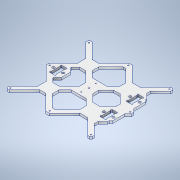
# Autodesk Inventor part: FROG
Saved by Autodesk Inventor 2023 (Build 270158000, 158)
## iProperties
Created: 2019-06-17
Part Number: FROG
Material: Aluminum 6061
Document SubType Name: Modeling
Designer: pepd9
Density: 2.7 g/cm^3
Appearance: Aluminum - Flat
Description: ALUM FROG
Author: pepd9
Autodesk Inventor part; units mm, degrees
ref_plane "YZ Plane" through (0, 0, 0) normal (1, 0, 0) x (0, 1, 0)
ref_plane "XZ Plane" through (0, 0, 0) normal (0, 1, 0) x (-1, 0, 0)
ref_plane "XY Plane" through (0, 0, 0) normal (0, 0, 1) x (1, 0, 0)
sketch "Sketch1" plane through (0, 0, 0) normal (0, 1, 0) x (-1, 0, 0)
  line L0 (-116, -3.7391) -> (-98.5, -21.2391)
  line L1 (-98.5, -21.2391) -> (-98.5, -52.5)
  line L2 (-98.5, -52.5) -> (-89, -62)
  line L3 (-89, -62) -> (-89, -75.5147)
  line L4 (-89, -75.5147) -> (-116, -102.5147)
  line L5 (-116, -102.5147) -> (-116, -107.4852)
  line L6 (-116, -107.4852) -> (-112.4852, -111)
  line L7 (-112.4852, -111) -> (-107.5147, -111)
  line L8 (-107.5147, -111) -> (-66.5147, -70)
  line L9 (-66.5147, -70) -> (-45.4001, -70)
  line L10 (-45.4001, -70) -> (-4.4001, -111)
  line L11 (-4.4001, -111) -> (4.4001, -111)
  line L12 (4.4001, -111) -> (45.4001, -70)
  line L13 (45.4001, -70) -> (61.5147, -70)
  line L14 (61.5147, -70) -> (102.5147, -111)
  line L15 (102.5147, -111) -> (107.4852, -111)
  line L16 (107.4852, -111) -> (111, -107.4852)
  line L17 (111, -107.4852) -> (111, -102.5147)
  line L18 (111, -102.5147) -> (73, -64.5147)
  line L19 (73, -64.5147) -> (73, -41.667)
  line L20 (73, -41.667) -> (111, -3.667)
  line L21 (111, -3.667) -> (111, 3.667)
  line L22 (111, 3.667) -> (73, 41.667)
  line L23 (73, 41.667) -> (73, 64.5147)
  line L24 (73, 64.5147) -> (111, 102.5147)
  line L25 (111, 102.5147) -> (111, 107.4852)
  line L26 (111, 107.4852) -> (107.4852, 111)
  line L27 (107.4852, 111) -> (102.5147, 111)
  line L28 (102.5147, 111) -> (61.5147, 70)
  line L29 (61.5147, 70) -> (45.4001, 70)
  line L30 (45.4001, 70) -> (4.4001, 111)
  line L31 (4.4001, 111) -> (-4.4001, 111)
  line L32 (-4.4001, 111) -> (-45.4001, 70)
  line L33 (-45.4001, 70) -> (-66.5147, 70)
  line L34 (-66.5147, 70) -> (-107.5147, 111)
  line L35 (-107.5147, 111) -> (-112.4852, 111)
  line L36 (-112.4852, 111) -> (-116, 107.4852)
  line L37 (-116, 107.4852) -> (-116, 102.5147)
  line L38 (-116, 102.5147) -> (-89, 75.5147)
  line L39 (-89, 75.5147) -> (-89, 62)
  line L40 (-89, 62) -> (-98.5, 52.5)
  line L41 (-98.5, 52.5) -> (-98.5, 21.2391)
  line L42 (-98.5, 21.2391) -> (-116, 3.7391)
  line L43 (-116, -3.7391) -> (-116, 3.7391)
  line L44 (-38.023, -28) -> (-18, -7.977)
  line L45 (-55, -28) -> (-38.023, -28)
  line L46 (-78.5, -4.5) -> (-55, -28)
  line L47 (-78.5, -4.5) -> (-78.5, 4.5)
  line L48 (-55, 28) -> (-78.5, 4.5)
  line L49 (-38.023, 28) -> (-55, 28)
  line L50 (-18, 7.977) -> (-38.023, 28)
  line L51 (-18, -7.977) -> (-18, 7.977)
  circle A0 centre (1.5, -19.5) radius 1.5
  circle A1 centre (1.5, 19.5) radius 1.5
  circle A2 centre (-110, 105) radius 1.5
  circle A3 centre (-93.5, 35) radius 1.6
  circle A4 centre (-93.5, -35) radius 1.6
  circle A5 centre (-73.5, 35) radius 1.6
  circle A6 centre (-73.5, -35) radius 1.6
  circle A7 centre (96.5, 0) radius 1.6
  circle A8 centre (76.5, 0) radius 1.6
  circle A9 centre (105, 0) radius 1.5
  circle A10 centre (0, 0) radius 1.5
  circle A11 centre (-110, 0) radius 1.5
  circle A12 centre (105, -105) radius 1.5
  circle A13 centre (-110, -105) radius 1.5
  circle A14 centre (105, 105) radius 1.5
  circle A15 centre (0, -105) radius 1.5
  circle A16 centre (0, 105) radius 1.5
  arc A17 (-89.1, -42.25) -> (-89.1, -48.25) centre (-89.1, -45.25) ccw
  line L52 (-89.1, -42.25) -> (-89, -42.25)
  line L53 (-88.5, -41.75) -> (-89, -42.25)
  line L54 (-88.5, -41.75) -> (-88.5, -28.25)
  line L55 (-89, -27.75) -> (-88.5, -28.25)
  line L56 (-89.1, -27.75) -> (-89, -27.75)
  arc A18 (-89.1, -21.75) -> (-89.1, -27.75) centre (-89.1, -24.75) ccw
  line L57 (-89.1, -21.75) -> (-77.9, -21.75)
  arc A19 (-77.9, -27.75) -> (-77.9, -21.75) centre (-77.9, -24.75) ccw
  line L58 (-77.9, -27.75) -> (-78, -27.75)
  line L59 (-78, -27.75) -> (-78.5, -28.25)
  line L60 (-78.5, -41.75) -> (-78.5, -28.25)
  line L61 (-78.5, -41.75) -> (-78, -42.25)
  line L62 (-77.9, -42.25) -> (-78, -42.25)
  arc A20 (-77.9, -48.25) -> (-77.9, -42.25) centre (-77.9, -45.25) ccw
  line L63 (-89.1, -48.25) -> (-77.9, -48.25)
  arc A21 (80.9, -7.25) -> (80.9, -13.25) centre (80.9, -10.25) ccw
  line L64 (80.9, -7.25) -> (81, -7.25)
  line L65 (81.5, -6.75) -> (81, -7.25)
  line L66 (81.5, -6.75) -> (81.5, 6.75)
  line L67 (81, 7.25) -> (81.5, 6.75)
  line L68 (80.9, 7.25) -> (81, 7.25)
  arc A22 (80.9, 13.25) -> (80.9, 7.25) centre (80.9, 10.25) ccw
  line L69 (80.9, 13.25) -> (92.1, 13.25)
  arc A23 (92.1, 7.25) -> (92.1, 13.25) centre (92.1, 10.25) ccw
  line L70 (92.1, 7.25) -> (92, 7.25)
  line L71 (92, 7.25) -> (91.5, 6.75)
  line L72 (91.5, -6.75) -> (91.5, 6.75)
  line L73 (91.5, -6.75) -> (92, -7.25)
  line L74 (92.1, -7.25) -> (92, -7.25)
  arc A24 (92.1, -13.25) -> (92.1, -7.25) centre (92.1, -10.25) ccw
  line L75 (80.9, -13.25) -> (92.1, -13.25)
  arc A25 (-89.1, 27.75) -> (-89.1, 21.75) centre (-89.1, 24.75) ccw
  line L76 (-89.1, 27.75) -> (-89, 27.75)
  line L77 (-88.5, 28.25) -> (-89, 27.75)
  line L78 (-88.5, 28.25) -> (-88.5, 41.75)
  line L79 (-89, 42.25) -> (-88.5, 41.75)
  line L80 (-89.1, 42.25) -> (-89, 42.25)
  arc A26 (-89.1, 48.25) -> (-89.1, 42.25) centre (-89.1, 45.25) ccw
  line L81 (-89.1, 48.25) -> (-77.9, 48.25)
  arc A27 (-77.9, 42.25) -> (-77.9, 48.25) centre (-77.9, 45.25) ccw
  line L82 (-77.9, 42.25) -> (-78, 42.25)
  line L83 (-78, 42.25) -> (-78.5, 41.75)
  line L84 (-78.5, 28.25) -> (-78.5, 41.75)
  line L85 (-78.5, 28.25) -> (-78, 27.75)
  line L86 (-77.9, 27.75) -> (-78, 27.75)
  arc A28 (-77.9, 21.75) -> (-77.9, 27.75) centre (-77.9, 24.75) ccw
  line L87 (-89.1, 21.75) -> (-77.9, 21.75)
  line L88 (3.6826, 94.747) -> (-3.6826, 94.7332)
  line L89 (36, 62.4296) -> (3.6826, 94.747)
  line L90 (36, 44.4853) -> (36, 62.4296)
  line L91 (19.5147, 28) -> (36, 44.4853)
  line L92 (-20.4337, 28) -> (19.5147, 28)
  line L93 (-37, 44.5663) -> (-20.4337, 28)
  line L94 (-37, 61.4158) -> (-37, 44.5663)
  line L95 (-3.6826, 94.7332) -> (-37, 61.4158)
  line L96 (-3.6826, -94.7332) -> (-37, -61.4158)
  line L97 (-37, -61.4158) -> (-37, -44.5663)
  line L98 (-37, -44.5663) -> (-20.4337, -28)
  line L99 (-20.4337, -28) -> (19.5147, -28)
  line L100 (19.5147, -28) -> (36, -44.4853)
  line L101 (36, -44.4853) -> (36, -62.4296)
  line L102 (36, -62.4296) -> (3.6826, -94.747)
  line L103 (3.6826, -94.747) -> (-3.6826, -94.7332)
  line L104 (17, -8.5147) -> (17, 8.5147)
  line L105 (17, 8.5147) -> (44.0147, 35.5294)
  line L106 (44.0147, 35.5294) -> (60.9853, 35.5294)
  line L107 (60.9853, 35.5294) -> (71.5, 25.0147)
  line L108 (71.5, -25.0147) -> (71.5, 25.0147)
  line L109 (71.5, -25.0147) -> (60.9853, -35.5294)
  line L110 (60.9853, -35.5294) -> (44.0147, -35.5294)
  line L111 (44.0147, -35.5294) -> (17, -8.5147)
  line L112 (-116, -111) -> (111, -111)
  line L113 (111, -111) -> (111, 111)
  line L114 (111, 111) -> (-116, 111)
  line L115 (-116, 111) -> (-116, -111)
  constraints: 232 end point, 29 centre point, 24 point on circle, 2 parallel, 1 horizontal, 1 perpendicular
sketch "Sketch2" plane through (0, 0, 0) normal (0, 1, 0) x (-1, 0, 0)
  circle A0 centre (105, -105) radius 1.5 projected
  circle A1 centre (0, -105) radius 1.5 projected
  circle A2 centre (-110, -105) radius 1.5 projected
  circle A3 centre (-110, 0) radius 1.5 projected
  circle A4 centre (0, 0) radius 1.5 projected
  circle A5 centre (105, 0) radius 1.5 projected
  circle A6 centre (105, 105) radius 1.5 projected
  circle A7 centre (-110, 105) radius 1.5 projected
  circle A8 centre (0, 105) radius 1.5 projected
  line L0 (102.5147, -111) -> (107.4852, -111) projected
  line L1 (111, -107.4852) -> (111, -102.5147) projected
  line L2 (-112.4852, -111) -> (-107.5147, -111) projected
  line L3 (-116, -102.5147) -> (-116, -107.4852) projected
  line L4 (-116, 107.4852) -> (-116, 102.5147) projected
  line L5 (-107.5147, 111) -> (-112.4852, 111) projected
  line L6 (107.4852, 111) -> (102.5147, 111) projected
  line L7 (111, 102.5147) -> (111, 107.4852) projected
  line L8 (111, 111) -> (-116, 111)
  line L9 (-116, 111) -> (-116, -111)
  line L10 (-116, -111) -> (111, -111)
  line L11 (111, -111) -> (111, 111)
  constraints: 8 end point, 2 parallel, 1 horizontal, 1 perpendicular
extrude "Extrusion1" add sketch "Sketch2" along normal blind 6.35
ref_plane "Work Plane1" through (2.5, 0, 111) normal (1, 0, 0) x (0, 0, -1)
sketch "Sketch6" plane through (0, 6.35, 0) normal (0, 1, 0) x (1, 0, 0)
  line L0 (73.5, -35) -> (93.5, -35)
  line L1 (73.5, 35) -> (93.5, 35)
  line L2 (80.75, 20.5) -> (94.25, 20.5)
  line L3 (94.25, 20.5) -> (94.25, 49.5)
  line L4 (94.25, 49.5) -> (80.75, 49.5)
  line L5 (80.75, 49.5) -> (80.75, 20.5)
  line L6 (80.75, 20.5) -> (94.25, 49.5) construction
  line L7 (94.25, 20.5) -> (80.75, 49.5) construction
  line L8 (80.75, -49.5) -> (94.25, -49.5)
  line L9 (94.25, -49.5) -> (94.25, -20.5)
  line L10 (94.25, -20.5) -> (80.75, -20.5)
  line L11 (80.75, -20.5) -> (80.75, -49.5)
  line L12 (80.75, -49.5) -> (94.25, -20.5) construction
  line L13 (94.25, -49.5) -> (80.75, -20.5) construction
  line L14 (87.5, -199.2866) -> (87.5, 58.81)
  line L15 (87.5, 0) -> (-102.0147, 0)
  line L16 (-75.75, 14.5) -> (-89.25, 14.5)
  line L17 (-89.25, 14.5) -> (-89.25, -14.5)
  line L18 (-89.25, -14.5) -> (-75.75, -14.5)
  line L19 (-75.75, -14.5) -> (-75.75, 14.5)
  line L20 (-75.75, 14.5) -> (-89.25, -14.5) construction
  line L21 (-89.25, 14.5) -> (-75.75, -14.5) construction
  point P0 (0, 0)
  point P1 (-82.5, 0)
  dimension "d16" = 13.5
  dimension "d17" = 29
  dimension "d18" = 13.5
  dimension "d19" = 29
  dimension "d39" = 6.75
  dimension "d40" = 6.75
  dimension "d67" = 87.5
  dimension "d68" = 13.5
  dimension "d69" = 29
  dimension "d70" = 170
  dimension "d76" = 14.5
  dimension "d77" = 14.5
  constraints: 44 end point, 6 horizontal, 6 parallel, 3 perpendicular, 2 midpoint, 2 point on line, 1 vertical
  measures "d16" distance of L4.end L3.end
  measures "d17" distance of L3.end L2.end
  measures "d18" distance of L10.end L9.end
  measures "d19" distance of L9.end L8.end
  measures "d39" distance between parallel lines of L14 L3
  measures "d40" distance between parallel lines of L14 L9
  measures "d67" distance from line of L14 point (0, 0)
  measures "d68" distance of L18.end L17.end
  measures "d69" distance of L17.end L16.end
  measures "d70" distance from line of L14 point (-82.5, 0)
  measures "d76" distance between parallel lines of L0 L8
  measures "d77" distance between parallel lines of L1 L4
extrude "Extrusion5" cut sketch "Sketch6" against normal through all
sketch "Sketch10" plane through (0, 6.35, 0) normal (0, 1, 0) x (1, 0, 0)
  line L0 (116, 111) -> (-111, 111) projected
  line L1 (-111, 111) -> (-111, -111) projected
  line L2 (-111, -111) -> (116, -111) projected
  line L3 (116, -111) -> (116, 111) projected
  circle A0 centre (0, -105) radius 1.5 projected
  circle A1 centre (-105, 105) radius 1.5 projected
  circle A2 centre (0, 105) radius 1.5 projected
  circle A3 centre (110, 105) radius 1.5 projected
  circle A4 centre (110, 0) radius 1.5 projected
  circle A5 centre (0, 0) radius 1.5 projected
  circle A6 centre (-105, 0) radius 1.5 projected
  circle A7 centre (-105, -105) radius 1.5 projected
  circle A8 centre (110, -105) radius 1.5 projected
  line L4 (94.25, -20.5) -> (94.25, -49.5) projected
  line L5 (80.75, -49.5) -> (80.75, -20.5) projected
  line L6 (80.75, 20.5) -> (80.75, 49.5) projected
  line L7 (94.25, 49.5) -> (94.25, 20.5) projected
  line L8 (80.75, -20.5) -> (94.25, -20.5) projected
  line L9 (94.25, -49.5) -> (80.75, -49.5) projected
  line L10 (80.75, 49.5) -> (94.25, 49.5) projected
  line L11 (94.25, 20.5) -> (80.75, 20.5) projected
extrude "Extrusion7" cut sketch "Sketch1" along normal blind 10 contours A0 | A1
sketch "Sketch13" plane through (0, 0, 0) normal (0, -1, 0) x (1, 0, 0)
  point P0 (0, 0)
extrude "Extrusion8" cut sketch "Sketch1" along normal blind 10 contours L6 L112 L115 | L115 L114 L36 | L8 L9 L10 L112 | L114 L32 L33 L34 | L12 L13 L14 L112 | L114 L28 L29 L30 | L16 L113 L112 | L114 L113 L26 | L18 L19 L20 L113 | L113 L22 L23 L24 | A0 | A1 | A2 | A9 | A10 | A11 | A12 | A13 | A14 | A15 | A16 | L89 L90 L91 L92 L93 L94 L95 L88 | L96 L97 L98 L99 L100 L101 L102 L103
sketch "Sketch14" plane through (0, 0, 0) normal (0, -1, 0) x (1, 0, 0)
  line L0 (89, -62) -> (89, -75.5147) projected
  line L1 (116, 102.5147) -> (89, 75.5147)
  line L2 (89, 75.5147) -> (89, 62)
  line L3 (89, 62) -> (107.1558, 43.8442)
  line L4 (107.1558, 43.8442) -> (107.1558, 12.5833)
  line L5 (98.5, 21.2391) -> (116, 3.7391) projected
  line L6 (107.1558, 12.5833) -> (116, 3.7391)
  line L7 (116, 107.4852) -> (116, -107.4852) projected
  line L8 (116, 0) -> (13.4853, 0)
  line L9 (116, -102.5147) -> (89, -75.5147)
  line L10 (89, -75.5147) -> (89, -62)
  line L11 (89, -62) -> (107.1558, -43.8442)
  line L12 (107.1558, -43.8442) -> (107.1558, -12.5833)
  line L13 (98.5, -21.2391) -> (116, -3.7391)
  line L14 (107.1558, -12.5833) -> (116, -3.7391)
  line L15 (116, 102.5147) -> (116, -102.5147)
  line L16 (55, 28) -> (78.5, 4.5) projected
  line L17 (38.023, 28) -> (55, 28) projected
  line L18 (18, 7.977) -> (38.023, 28) projected
  line L19 (18, -7.977) -> (18, 7.977) projected
  line L20 (38.023, -28) -> (18, -7.977) projected
  line L21 (55, -28) -> (38.023, -28) projected
  line L22 (78.5, -4.5) -> (55, -28) projected
  line L23 (78.5, -4.5) -> (78.5, 4.5) projected
  point P0 (0, 0)
  constraints: 26 end point, 3 symmetric about line, 2 point on line, 1 collinear, 1 horizontal, 1 midpoint, 1 parallel, 1 vertical
extrude "Extrusion9" cut sketch "Sketch14" against normal blind 10
sketch "Sketch15" plane through (0, 0, 0) normal (0, -1, 0) x (1, 0, 0)
  line L0 (-17, -8.5147) -> (-17, 8.5147) projected
  line L1 (-17, 8.5147) -> (-44.0147, 35.5294) projected
  line L2 (-44.0147, 35.5294) -> (-60.9853, 35.5294) projected
  line L3 (-60.9853, 35.5294) -> (-71.5, 25.0147) projected
  line L4 (-44.0147, -35.5294) -> (-17, -8.5147) projected
  line L5 (-60.9853, -35.5294) -> (-44.0147, -35.5294) projected
  line L6 (107.1558, -12.5833) -> (116, -3.7391) projected
  line L7 (116, 3.7391) -> (116, -3.7391) projected
  line L8 (116, 3.7391) -> (107.1558, 12.5833) projected
  line L9 (107.1558, 12.5833) -> (107.1558, 43.8442) projected
  line L10 (107.1558, 43.8442) -> (89, 62) projected
  line L11 (89, 62) -> (89, 75.5147) projected
  line L12 (89, 75.5147) -> (116, 102.5147) projected
  line L13 (116, 107.4852) -> (116, 102.5147) projected
  line L14 (116, 107.4852) -> (112.4852, 111) projected
  line L15 (107.5147, 111) -> (112.4852, 111) projected
  line L16 (107.5147, 111) -> (66.5147, 70) projected
  line L17 (66.5147, 70) -> (45.4001, 70) projected
  line L18 (45.4001, 70) -> (4.4001, 111) projected
  line L19 (-4.4001, 111) -> (4.4001, 111) projected
  line L20 (-4.4001, 111) -> (-45.4001, 70) projected
  line L21 (-45.4001, 70) -> (-61.5147, 70) projected
  line L22 (-61.5147, 70) -> (-102.5147, 111) projected
  line L23 (-107.4852, 111) -> (-102.5147, 111) projected
  line L24 (-107.4852, 111) -> (-111, 107.4852) projected
  line L25 (-111, 102.5147) -> (-111, 107.4852) projected
  line L26 (-111, 102.5147) -> (-73, 64.5147) projected
  line L27 (-73, 64.5147) -> (-73, 41.667) projected
  line L28 (-73, 41.667) -> (-111, 3.667) projected
  line L29 (-111, -3.667) -> (-111, 3.667) projected
  line L30 (-111, -3.667) -> (-73, -41.667) projected
  line L31 (-73, -41.667) -> (-73, -64.5147) projected
  line L32 (-73, -64.5147) -> (-111, -102.5147) projected
  line L33 (-111, -107.4852) -> (-111, -102.5147) projected
  line L34 (-111, -107.4852) -> (-107.4852, -111) projected
  line L35 (-102.5147, -111) -> (-107.4852, -111) projected
  line L36 (-102.5147, -111) -> (-61.5147, -70) projected
  line L37 (-61.5147, -70) -> (-45.4001, -70) projected
  line L38 (-45.4001, -70) -> (-4.4001, -111) projected
  line L39 (4.4001, -111) -> (-4.4001, -111) projected
  line L40 (4.4001, -111) -> (45.4001, -70) projected
  line L41 (45.4001, -70) -> (66.5147, -70) projected
  line L42 (66.5147, -70) -> (107.5147, -111) projected
  line L43 (112.4852, -111) -> (107.5147, -111) projected
  line L44 (112.4852, -111) -> (116, -107.4852) projected
  line L45 (116, -102.5147) -> (116, -107.4852) projected
  line L46 (116, -102.5147) -> (89, -75.5147) projected
  line L47 (89, -75.5147) -> (89, -62) projected
  line L48 (89, -62) -> (107.1558, -43.8442) projected
  line L49 (107.1558, -43.8442) -> (107.1558, -12.5833) projected
  line L50 (18, -7.977) -> (18, 7.977) projected
  line L51 (18, 7.977) -> (38.023, 28) projected
  line L52 (38.023, 28) -> (55, 28) projected
  line L53 (55, 28) -> (78.5, 4.5) projected
  line L54 (78.5, 4.5) -> (78.5, -4.5) projected
  line L55 (78.5, -4.5) -> (55, -28) projected
  line L56 (55, -28) -> (38.023, -28) projected
  line L57 (38.023, -28) -> (18, -7.977) projected
  line L58 (94.25, -20.5) -> (94.25, -49.5) projected
  line L59 (37, -61.4158) -> (3.6826, -94.7332) projected
  line L60 (3.6826, -94.7332) -> (-3.6826, -94.747) projected
  line L61 (-3.6826, -94.747) -> (-36, -62.4296) projected
  line L62 (-36, -62.4296) -> (-36, -44.4853) projected
  line L63 (-36, -44.4853) -> (-19.5147, -28) projected
  line L64 (-19.5147, -28) -> (20.4337, -28) projected
  line L65 (20.4337, -28) -> (37, -44.5663) projected
  line L66 (37, -44.5663) -> (37, -61.4158) projected
  line L67 (3.6826, 94.7332) -> (37, 61.4158) projected
  line L68 (37, 61.4158) -> (37, 44.5663) projected
  line L69 (37, 44.5663) -> (20.4337, 28) projected
  line L70 (20.4337, 28) -> (-19.5147, 28) projected
  line L71 (-19.5147, 28) -> (-36, 44.4853) projected
  line L72 (-36, 44.4853) -> (-36, 62.4296) projected
  line L73 (-36, 62.4296) -> (-3.6826, 94.747) projected
  line L74 (-3.6826, 94.747) -> (3.6826, 94.7332) projected
  circle A0 centre (-1.5, -19.5) radius 1.5 projected
  circle A1 centre (-1.5, 19.5) radius 1.5 projected
  circle A2 centre (110, 105) radius 1.5 projected
  circle A3 centre (-105, 105) radius 1.5 projected
  circle A4 centre (-105, 0) radius 1.5 projected
  circle A5 centre (0, 0) radius 1.5 projected
  circle A6 centre (110, 0) radius 1.5 projected
  circle A7 centre (110, -105) radius 1.5 projected
  circle A8 centre (0, -105) radius 1.5 projected
  circle A9 centre (-105, -105) radius 1.5 projected
  circle A10 centre (0, 105) radius 1.5 projected
  line L75 (94.25, 49.5) -> (94.25, 20.5) projected
  line L76 (-71.5, -25.0147) -> (-60.9853, -35.5294) projected
  line L77 (-71.5, -25.0147) -> (-71.5, 25.0147) projected
  line L78 (-71.5, 22.197) -> (-61.803, 12.5)
  line L79 (-61.803, 12.5) -> (-61.803, -12.5)
  line L80 (-61.803, -12.5) -> (-71.5, -22.197)
  line L81 (80.75, -49.5) -> (80.75, -20.5) projected
  line L82 (80.75, 20.5) -> (80.75, 49.5) projected
  line L83 (94.25, -49.5) -> (80.75, -49.5) projected
  line L84 (80.75, -20.5) -> (94.25, -20.5) projected
  line L85 (80.75, 49.5) -> (94.25, 49.5) projected
  line L86 (94.25, 20.5) -> (80.75, 20.5) projected
  dimension "d57" = 25
  constraints: 6 end point, 2 parallel, 2 point on line, 1 vertical
  measures "d57" distance of L78.end L79.end
extrude "Extrusion10" cut sketch "Sketch15" against normal blind 10 contours L4 L5 L76 L77 L80 L79 L78 L3 L2 L1 L0
sketch "Sketch17" plane through (0, 6.35, 0) normal (0, 1, 0) x (1, 0, 0)
  line L0 (89, 62) -> (107.1558, 43.8442) projected
  line L1 (102.1558, 48.8442) -> (102.1558, 51.8442)
  line L2 (102.1558, 51.8442) -> (89, 65)
  line L3 (89, 62) -> (89, 75.5147) projected
  line L4 (107.1558, -43.8442) -> (89, -62) projected
  line L5 (102.1558, -48.8442) -> (102.1558, -51.8442)
  line L6 (102.1558, -51.8442) -> (89, -65)
  line L7 (89, -75.5147) -> (89, -62) projected
  line L8 (107.1558, -43.8442) -> (107.1558, -12.5833) projected
  point P0 (0, 0)
  dimension "d61" = 5
  dimension "d62" = 3
  dimension "d63" = 5
  dimension "d64" = 3
  constraints: 8 end point, 4 point on line, 2 parallel, 2 vertical
  measures "d61" distance from line of L1 L0.end
  measures "d62" distance of L1.start L1.end
  measures "d63" distance between parallel lines of L8 L5
  measures "d64" distance of L5.start L5.end
extrude "Extrusion11" add sketch "Sketch17" against normal up to surface (6.35 mm away)
sketch "Sketch19" plane through (0, 6.35, 0) normal (0, 1, 0) x (1, 0, 0)
  line L0 (94.25, -49.5) -> (80.75, -49.5) construction
  line L1 (94.25, -48) -> (80.75, -48)
  line L2 (80.75, -51) -> (94.25, -51)
  arc A0 (94.25, -51) -> (94.25, -48) centre (94.25, -49.5) ccw
  arc A1 (80.75, -48) -> (80.75, -51) centre (80.75, -49.5) ccw
  line L3 (80.75, -20.5) -> (94.25, -20.5) projected
  line L4 (94.25, -20.5) -> (80.75, -20.5) projected
  line L5 (94.25, -20.5) -> (80.75, -20.5) construction
  line L6 (94.25, -19) -> (80.75, -19)
  line L7 (80.75, -22) -> (94.25, -22)
  arc A2 (94.25, -22) -> (94.25, -19) centre (94.25, -20.5) ccw
  arc A3 (80.75, -19) -> (80.75, -22) centre (80.75, -20.5) ccw
  line L8 (-75.75, -14.5) -> (-89.25, -14.5) construction
  line L9 (-75.75, -13) -> (-89.25, -13)
  line L10 (-89.25, -16) -> (-75.75, -16)
  arc A4 (-75.75, -16) -> (-75.75, -13) centre (-75.75, -14.5) ccw
  arc A5 (-89.25, -13) -> (-89.25, -16) centre (-89.25, -14.5) ccw
  line L11 (-75.75, -14.5) -> (-75.75, 14.5) projected
  line L12 (-75.75, 14.5) -> (-89.25, 14.5) construction
  line L13 (-75.75, 16) -> (-89.25, 16)
  line L14 (-89.25, 13) -> (-75.75, 13)
  arc A6 (-75.75, 13) -> (-75.75, 16) centre (-75.75, 14.5) ccw
  arc A7 (-89.25, 16) -> (-89.25, 13) centre (-89.25, 14.5) ccw
  line L15 (94.25, 20.5) -> (80.75, 20.5) projected
  line L16 (94.25, 20.5) -> (80.75, 20.5) construction
  line L17 (94.25, 22) -> (80.75, 22)
  line L18 (80.75, 19) -> (94.25, 19)
  arc A8 (94.25, 19) -> (94.25, 22) centre (94.25, 20.5) ccw
  arc A9 (80.75, 22) -> (80.75, 19) centre (80.75, 20.5) ccw
  line L19 (80.75, 49.5) -> (94.25, 49.5) projected
  line L20 (94.25, 49.5) -> (80.75, 49.5) construction
  line L21 (94.25, 51) -> (80.75, 51)
  line L22 (80.75, 48) -> (94.25, 48)
  arc A10 (94.25, 48) -> (94.25, 51) centre (94.25, 49.5) ccw
  arc A11 (80.75, 51) -> (80.75, 48) centre (80.75, 49.5) ccw
  point P0 (87.5, -49.5)
  point P1 (87.5, -20.5)
  point P2 (-82.5, -14.5)
  point P3 (-82.5, 14.5)
  point P4 (87.5, 20.5)
  point P5 (87.5, 49.5)
  dimension "d71" = 3
  dimension "d75" = 3
  dimension "d81" = 3
  dimension "d82" = 3
  dimension "d84" = 3
  dimension "d85" = 3
  constraints: 48 end point, 24 point on circle, 24 tangent, 12 centre point, 9 equal length, 6 midpoint, 2 horizontal, 1 perpendicular
  measures "d71" diameter of A1
  measures "d75" diameter of A3
  measures "d81" diameter of A5
  measures "d82" diameter of A7
  measures "d84" diameter of A9
  measures "d85" diameter of A11
extrude "Extrusion12" cut sketch "Sketch19" against normal through all
fillet "Fillet1" radius 2 4 edges at (94.25, 3.175, 48) (80.75, 3.175, 48) (94.25, 3.175, 22) (80.75, 3.175, 22)
fillet "Fillet2" radius 2 8 edges at (-89.25, 3.175, -13) (-75.75, 3.175, -13) (-89.25, 3.175, 13) (-75.75, 3.175, 13) (94.25, 3.175, -22) (94.25, 3.175, -48) (80.75, 3.175, -48) (80.75, 3.175, -22)
sketch "Sketch20" plane through (0, 6.35, 0) normal (0, 1, 0) x (1, 0, 0)
  line L0 (94.25, -51) -> (80.75, -51) projected
  line L1 (87.5, -51) -> (87.5, -41.5459)
  line L2 (94.25, 19) -> (80.75, 19) projected
  point P0 (0, 0)
  point P1 (100.2, -35)
  point P2 (74.8, -35)
  point P3 (100.2, 35)
  point P4 (74.8, 35)
  point P5 (-69.8, 0)
  point P6 (-95.2, 0)
  dimension "d86" = 25.4
  dimension "d87" = 12.7
  dimension "d88" = 16
  dimension "d89" = 25.4
  dimension "d90" = 12.7
  dimension "d91" = 16
  dimension "d92" = 25.4
  dimension "d93" = 182.7
  constraints: 3 horizontal alignment, 2 end point, 1 midpoint, 1 vertical
  measures "d86" distance of point (100.2, -35) point (74.8, -35)
  measures "d87" distance from line of L1 point (74.8, -35)
  measures "d88" distance from line of L0 point (74.8, -35)
  measures "d89" distance of point (100.2, 35) point (74.8, 35)
  measures "d90" distance from line of L1 point (74.8, 35)
  measures "d91" distance from line of L2 point (74.8, 35)
  measures "d92" distance of point (-95.2, 0) point (-69.8, 0)
  measures "d93" distance from line of L1 point (-95.2, 0)
hole "Hole3" at (100.2, 6.35, 35) at (74.8, 6.35, 35) at (100.2, 6.35, -35) at (74.8, 6.35, -35) at (-69.8, 6.35, 0) at (-95.2, 6.35, 0) direction (0, -1, 0) diameter 6.6 end through all
sketch "Waterjet Sketch" plane through (0, 6.35, 0) normal (0, 1, 0) x (1, 0, 0)
  circle A0 centre (-69.8, 0) radius 3.3 projected
  circle A1 centre (100.2, 35) radius 3.3 projected
  circle A2 centre (100.2, -35) radius 3.3 projected
  circle A3 centre (74.8, -35) radius 3.3 projected
  circle A4 centre (74.8, 35) radius 3.3 projected
  circle A5 centre (-95.2, 0) radius 3.3 projected
  line L0 (18, -7.977) -> (18, 7.977) projected
  line L1 (18, 7.977) -> (38.023, 28) projected
  line L2 (38.023, 28) -> (55, 28) projected
  line L3 (55, 28) -> (78.5, 4.5) projected
  line L4 (78.5, 4.5) -> (78.5, -4.5) projected
  line L5 (78.5, -4.5) -> (55, -28) projected
  line L6 (55, -28) -> (38.023, -28) projected
  line L7 (38.023, -28) -> (18, -7.977) projected
  line L8 (116, 3.7391) -> (107.1558, 12.5833) projected
  line L9 (107.1558, 12.5833) -> (107.1558, 43.8442) projected
  line L10 (107.1558, 43.8442) -> (102.1558, 48.8442) projected
  line L11 (102.1558, 48.8442) -> (102.1558, 51.8442) projected
  line L12 (102.1558, 51.8442) -> (89, 65) projected
  line L13 (89, 65) -> (89, 75.5147) projected
  line L14 (89, 75.5147) -> (116, 102.5147) projected
  line L15 (116, 102.5147) -> (116, 107.4852) projected
  line L16 (116, 107.4852) -> (112.4852, 111) projected
  line L17 (112.4852, 111) -> (107.5147, 111) projected
  line L18 (107.5147, 111) -> (66.5147, 70) projected
  line L19 (66.5147, 70) -> (45.4001, 70) projected
  line L20 (45.4001, 70) -> (4.4001, 111) projected
  line L21 (4.4001, 111) -> (-4.4001, 111) projected
  line L22 (-4.4001, 111) -> (-45.4001, 70) projected
  line L23 (-45.4001, 70) -> (-61.5147, 70) projected
  line L24 (-61.5147, 70) -> (-102.5147, 111) projected
  line L25 (-102.5147, 111) -> (-107.4852, 111) projected
  line L26 (-107.4852, 111) -> (-111, 107.4852) projected
  line L27 (-111, 107.4852) -> (-111, 102.5147) projected
  line L28 (-111, 102.5147) -> (-73, 64.5147) projected
  line L29 (-73, 64.5147) -> (-73, 41.667) projected
  line L30 (-73, 41.667) -> (-111, 3.667) projected
  line L31 (-111, 3.667) -> (-111, -3.667) projected
  line L32 (-111, -3.667) -> (-73, -41.667) projected
  line L33 (-73, -41.667) -> (-73, -64.5147) projected
  line L34 (-73, -64.5147) -> (-111, -102.5147) projected
  line L35 (-111, -102.5147) -> (-111, -107.4852) projected
  line L36 (-111, -107.4852) -> (-107.4852, -111) projected
  line L37 (-107.4852, -111) -> (-102.5147, -111) projected
  line L38 (-102.5147, -111) -> (-61.5147, -70) projected
  line L39 (-61.5147, -70) -> (-45.4001, -70) projected
  line L40 (-45.4001, -70) -> (-4.4001, -111) projected
  line L41 (-4.4001, -111) -> (4.4001, -111) projected
  line L42 (4.4001, -111) -> (45.4001, -70) projected
  line L43 (45.4001, -70) -> (66.5147, -70) projected
  line L44 (66.5147, -70) -> (107.5147, -111) projected
  line L45 (107.5147, -111) -> (112.4852, -111) projected
  line L46 (112.4852, -111) -> (116, -107.4852) projected
  line L47 (116, -107.4852) -> (116, -102.5147) projected
  line L48 (116, -102.5147) -> (89, -75.5147) projected
  line L49 (89, -75.5147) -> (89, -65) projected
  line L50 (89, -65) -> (102.1558, -51.8442) projected
  line L51 (102.1558, -51.8442) -> (102.1558, -48.8442) projected
  line L52 (102.1558, -48.8442) -> (107.1558, -43.8442) projected
  line L53 (107.1558, -43.8442) -> (107.1558, -12.5833) projected
  line L54 (107.1558, -12.5833) -> (116, -3.7391) projected
  line L55 (116, -3.7391) -> (116, 3.7391) projected
  line L56 (-36, -44.4853) -> (-19.5147, -28) projected
  line L57 (-19.5147, -28) -> (20.4337, -28) projected
  line L58 (20.4337, -28) -> (37, -44.5663) projected
  line L59 (37, -44.5663) -> (37, -61.4158) projected
  line L60 (37, -61.4158) -> (3.6826, -94.7332) projected
  line L61 (3.6826, -94.7332) -> (-3.6826, -94.747) projected
  line L62 (-3.6826, -94.747) -> (-36, -62.4296) projected
  line L63 (-36, -62.4296) -> (-36, -44.4853) projected
  line L64 (-19.5147, 28) -> (-36, 44.4853) projected
  line L65 (-36, 44.4853) -> (-36, 62.4296) projected
  line L66 (-36, 62.4296) -> (-3.6826, 94.747) projected
  line L67 (-3.6826, 94.747) -> (3.6826, 94.7332) projected
  line L68 (3.6826, 94.7332) -> (37, 61.4158) projected
  line L69 (37, 61.4158) -> (37, 44.5663) projected
  line L70 (37, 44.5663) -> (20.4337, 28) projected
  line L71 (20.4337, 28) -> (-19.5147, 28) projected
  circle A6 centre (-1.5, 19.5) radius 1.5 projected
  circle A7 centre (-1.5, -19.5) radius 1.5 projected
  circle A8 centre (0, -105) radius 1.5 projected
  circle A9 centre (-105, 105) radius 1.5 projected
  circle A10 centre (0, 105) radius 1.5 projected
  circle A11 centre (110, 105) radius 1.5 projected
  circle A12 centre (110, 0) radius 1.5 projected
  circle A13 centre (0, 0) radius 1.5 projected
  circle A14 centre (-105, 0) radius 1.5 projected
  circle A15 centre (-105, -105) radius 1.5 projected
  circle A16 centre (110, -105) radius 1.5 projected
  line L72 (-17, 8.5147) -> (-17, -8.5147) projected
  line L73 (-17, -8.5147) -> (-44.0147, -35.5294) projected
  line L74 (-44.0147, -35.5294) -> (-60.9853, -35.5294) projected
  line L75 (-60.9853, -35.5294) -> (-71.5, -25.0147) projected
  line L76 (-71.5, -25.0147) -> (-71.5, -22.197) projected
  line L77 (-71.5, -22.197) -> (-61.803, -12.5) projected
  line L78 (-61.803, -12.5) -> (-61.803, 12.5) projected
  line L79 (-61.803, 12.5) -> (-71.5, 22.197) projected
  line L80 (-71.5, 22.197) -> (-71.5, 25.0147) projected
  line L81 (-71.5, 25.0147) -> (-60.9853, 35.5294) projected
  line L82 (-60.9853, 35.5294) -> (-44.0147, 35.5294) projected
  line L83 (-44.0147, 35.5294) -> (-17, 8.5147) projected
  arc A17 (79.8929, 21.731) -> (80.75, 23.3723) centre (78.75, 23.3723) ccw projected
  line L84 (80.75, 23.3723) -> (80.75, 46.6277) projected
  arc A18 (80.75, 46.6277) -> (79.8929, 48.269) centre (78.75, 46.6277) ccw projected
  arc A19 (80.75, 51) -> (79.8929, 48.269) centre (80.75, 49.5) ccw projected
  line L85 (80.75, 51) -> (94.25, 51) projected
  arc A20 (95.1071, 48.269) -> (94.25, 51) centre (94.25, 49.5) ccw projected
  arc A21 (95.1071, 48.269) -> (94.25, 46.6277) centre (96.25, 46.6277) ccw projected
  line L86 (94.25, 46.6277) -> (94.25, 23.3723) projected
  arc A22 (94.25, 23.3723) -> (95.1071, 21.731) centre (96.25, 23.3723) ccw projected
  arc A23 (94.25, 19) -> (95.1071, 21.731) centre (94.25, 20.5) ccw projected
  line L87 (94.25, 19) -> (80.75, 19) projected
  arc A24 (79.8929, 21.731) -> (80.75, 19) centre (80.75, 20.5) ccw projected
  arc A25 (80.75, -23.3723) -> (79.8929, -21.731) centre (78.75, -23.3723) ccw projected
  arc A26 (80.75, -19) -> (79.8929, -21.731) centre (80.75, -20.5) ccw projected
  line L88 (80.75, -19) -> (94.25, -19) projected
  arc A27 (95.1071, -21.731) -> (94.25, -19) centre (94.25, -20.5) ccw projected
  arc A28 (95.1071, -21.731) -> (94.25, -23.3723) centre (96.25, -23.3723) ccw projected
  line L89 (94.25, -23.3723) -> (94.25, -46.6277) projected
  arc A29 (94.25, -46.6277) -> (95.1071, -48.269) centre (96.25, -46.6277) ccw projected
  arc A30 (94.25, -51) -> (95.1071, -48.269) centre (94.25, -49.5) ccw projected
  line L90 (94.25, -51) -> (80.75, -51) projected
  arc A31 (79.8929, -48.269) -> (80.75, -51) centre (80.75, -49.5) ccw projected
  arc A32 (79.8929, -48.269) -> (80.75, -46.6277) centre (78.75, -46.6277) ccw projected
  line L91 (80.75, -46.6277) -> (80.75, -23.3723) projected
  arc A33 (-75.75, -11.6277) -> (-74.8929, -13.269) centre (-73.75, -11.6277) ccw projected
  arc A34 (-75.75, -16) -> (-74.8929, -13.269) centre (-75.75, -14.5) ccw projected
  line L92 (-75.75, -16) -> (-89.25, -16) projected
  arc A35 (-90.1071, -13.269) -> (-89.25, -16) centre (-89.25, -14.5) ccw projected
  arc A36 (-90.1071, -13.269) -> (-89.25, -11.6277) centre (-91.25, -11.6277) ccw projected
  line L93 (-89.25, -11.6277) -> (-89.25, 11.6277) projected
  arc A37 (-89.25, 11.6277) -> (-90.1071, 13.269) centre (-91.25, 11.6277) ccw projected
  arc A38 (-89.25, 16) -> (-90.1071, 13.269) centre (-89.25, 14.5) ccw projected
  line L94 (-89.25, 16) -> (-75.75, 16) projected
  arc A39 (-74.8929, 13.269) -> (-75.75, 16) centre (-75.75, 14.5) ccw projected
  arc A40 (-74.8929, 13.269) -> (-75.75, 11.6277) centre (-73.75, 11.6277) ccw projected
  line L95 (-75.75, 11.6277) -> (-75.75, -11.6277) projected
sketch "Sketch23" plane through (0, 6.35, 0) normal (0, 1, 0) x (1, 0, 0)
  circle A0 centre (-69.8, 0) radius 3.3 projected
  circle A1 centre (100.2, 35) radius 3.3 projected
  circle A2 centre (100.2, -35) radius 3.3 projected
  circle A3 centre (74.8, -35) radius 3.3 projected
  circle A4 centre (74.8, 35) radius 3.3 projected
  circle A5 centre (-95.2, 0) radius 3.3 projected
  line L0 (18, -7.977) -> (18, 7.977) projected
  line L1 (18, 7.977) -> (38.023, 28) projected
  line L2 (38.023, 28) -> (55, 28) projected
  line L3 (55, 28) -> (78.5, 4.5) projected
  line L4 (78.5, 4.5) -> (78.5, -4.5) projected
  line L5 (78.5, -4.5) -> (55, -28) projected
  line L6 (55, -28) -> (38.023, -28) projected
  line L7 (38.023, -28) -> (18, -7.977) projected
  line L8 (116, 3.7391) -> (107.1558, 12.5833) projected
  line L9 (107.1558, 12.5833) -> (107.1558, 43.8442) projected
  line L10 (107.1558, 43.8442) -> (102.1558, 48.8442) projected
  line L11 (102.1558, 48.8442) -> (102.1558, 51.8442) projected
  line L12 (102.1558, 51.8442) -> (89, 65) projected
  line L13 (89, 65) -> (89, 75.5147) projected
  line L14 (89, 75.5147) -> (116, 102.5147) projected
  line L15 (116, 102.5147) -> (116, 107.4852) projected
  line L16 (116, 107.4852) -> (112.4852, 111) projected
  line L17 (112.4852, 111) -> (107.5147, 111) projected
  line L18 (107.5147, 111) -> (66.5147, 70) projected
  line L19 (66.5147, 70) -> (45.4001, 70) projected
  line L20 (45.4001, 70) -> (4.4001, 111) projected
  line L21 (4.4001, 111) -> (-4.4001, 111) projected
  line L22 (-4.4001, 111) -> (-45.4001, 70) projected
  line L23 (-45.4001, 70) -> (-61.5147, 70) projected
  line L24 (-61.5147, 70) -> (-102.5147, 111) projected
  line L25 (-102.5147, 111) -> (-107.4852, 111) projected
  line L26 (-107.4852, 111) -> (-111, 107.4852) projected
  line L27 (-111, 107.4852) -> (-111, 102.5147) projected
  line L28 (-111, 102.5147) -> (-73, 64.5147) projected
  line L29 (-73, 64.5147) -> (-73, 41.667) projected
  line L30 (-73, 41.667) -> (-111, 3.667) projected
  line L31 (-111, 3.667) -> (-111, -3.667) projected
  line L32 (-111, -3.667) -> (-73, -41.667) projected
  line L33 (-73, -41.667) -> (-73, -64.5147) projected
  line L34 (-73, -64.5147) -> (-111, -102.5147) projected
  line L35 (-111, -102.5147) -> (-111, -107.4852) projected
  line L36 (-111, -107.4852) -> (-107.4852, -111) projected
  line L37 (-107.4852, -111) -> (-102.5147, -111) projected
  line L38 (-102.5147, -111) -> (-61.5147, -70) projected
  line L39 (-61.5147, -70) -> (-45.4001, -70) projected
  line L40 (-45.4001, -70) -> (-4.4001, -111) projected
  line L41 (-4.4001, -111) -> (4.4001, -111) projected
  line L42 (4.4001, -111) -> (45.4001, -70) projected
  line L43 (45.4001, -70) -> (66.5147, -70) projected
  line L44 (66.5147, -70) -> (107.5147, -111) projected
  line L45 (107.5147, -111) -> (112.4852, -111) projected
  line L46 (112.4852, -111) -> (116, -107.4852) projected
  line L47 (116, -107.4852) -> (116, -102.5147) projected
  line L48 (116, -102.5147) -> (89, -75.5147) projected
  line L49 (89, -75.5147) -> (89, -65) projected
  line L50 (89, -65) -> (102.1558, -51.8442) projected
  line L51 (102.1558, -51.8442) -> (102.1558, -48.8442) projected
  line L52 (102.1558, -48.8442) -> (107.1558, -43.8442) projected
  line L53 (107.1558, -43.8442) -> (107.1558, -12.5833) projected
  line L54 (107.1558, -12.5833) -> (116, -3.7391) projected
  line L55 (116, -3.7391) -> (116, 3.7391) projected
  line L56 (-36, -44.4853) -> (-19.5147, -28) projected
  line L57 (-19.5147, -28) -> (20.4337, -28) projected
  line L58 (20.4337, -28) -> (37, -44.5663) projected
  line L59 (37, -44.5663) -> (37, -61.4158) projected
  line L60 (37, -61.4158) -> (3.6826, -94.7332) projected
  line L61 (3.6826, -94.7332) -> (-3.6826, -94.747) projected
  line L62 (-3.6826, -94.747) -> (-36, -62.4296) projected
  line L63 (-36, -62.4296) -> (-36, -44.4853) projected
  line L64 (-19.5147, 28) -> (-36, 44.4853) projected
  line L65 (-36, 44.4853) -> (-36, 62.4296) projected
  line L66 (-36, 62.4296) -> (-3.6826, 94.747) projected
  line L67 (-3.6826, 94.747) -> (3.6826, 94.7332) projected
  line L68 (3.6826, 94.7332) -> (37, 61.4158) projected
  line L69 (37, 61.4158) -> (37, 44.5663) projected
  line L70 (37, 44.5663) -> (20.4337, 28) projected
  line L71 (20.4337, 28) -> (-19.5147, 28) projected
  circle A6 centre (-1.5, 19.5) radius 1.5 projected
  circle A7 centre (-1.5, -19.5) radius 1.5 projected
  circle A8 centre (0, -105) radius 1.5 projected
  circle A9 centre (-105, 105) radius 1.5 projected
  circle A10 centre (0, 105) radius 1.5 projected
  circle A11 centre (110, 105) radius 1.5 projected
  circle A12 centre (110, 0) radius 1.5 projected
  circle A13 centre (0, 0) radius 1.5 projected
  circle A14 centre (-105, 0) radius 1.5 projected
  circle A15 centre (-105, -105) radius 1.5 projected
  circle A16 centre (110, -105) radius 1.5 projected
  line L72 (-17, 8.5147) -> (-17, -8.5147) projected
  line L73 (-17, -8.5147) -> (-44.0147, -35.5294) projected
  line L74 (-44.0147, -35.5294) -> (-60.9853, -35.5294) projected
  line L75 (-60.9853, -35.5294) -> (-71.5, -25.0147) projected
  line L76 (-71.5, -25.0147) -> (-71.5, -22.197) projected
  line L77 (-71.5, -22.197) -> (-61.803, -12.5) projected
  line L78 (-61.803, -12.5) -> (-61.803, 12.5) projected
  line L79 (-61.803, 12.5) -> (-71.5, 22.197) projected
  line L80 (-71.5, 22.197) -> (-71.5, 25.0147) projected
  line L81 (-71.5, 25.0147) -> (-60.9853, 35.5294) projected
  line L82 (-60.9853, 35.5294) -> (-44.0147, 35.5294) projected
  line L83 (-44.0147, 35.5294) -> (-17, 8.5147) projected
  arc A17 (79.8929, 21.731) -> (80.75, 23.3723) centre (78.75, 23.3723) ccw projected
  line L84 (80.75, 23.3723) -> (80.75, 46.6277) projected
  arc A18 (80.75, 46.6277) -> (79.8929, 48.269) centre (78.75, 46.6277) ccw projected
  arc A19 (80.75, 51) -> (79.8929, 48.269) centre (80.75, 49.5) ccw projected
  line L85 (80.75, 51) -> (94.25, 51) projected
  arc A20 (95.1071, 48.269) -> (94.25, 51) centre (94.25, 49.5) ccw projected
  arc A21 (95.1071, 48.269) -> (94.25, 46.6277) centre (96.25, 46.6277) ccw projected
  line L86 (94.25, 46.6277) -> (94.25, 23.3723) projected
  arc A22 (94.25, 23.3723) -> (95.1071, 21.731) centre (96.25, 23.3723) ccw projected
  arc A23 (94.25, 19) -> (95.1071, 21.731) centre (94.25, 20.5) ccw projected
  line L87 (94.25, 19) -> (80.75, 19) projected
  arc A24 (79.8929, 21.731) -> (80.75, 19) centre (80.75, 20.5) ccw projected
  arc A25 (80.75, -23.3723) -> (79.8929, -21.731) centre (78.75, -23.3723) ccw projected
  arc A26 (80.75, -19) -> (79.8929, -21.731) centre (80.75, -20.5) ccw projected
  line L88 (80.75, -19) -> (94.25, -19) projected
  arc A27 (95.1071, -21.731) -> (94.25, -19) centre (94.25, -20.5) ccw projected
  arc A28 (95.1071, -21.731) -> (94.25, -23.3723) centre (96.25, -23.3723) ccw projected
  line L89 (94.25, -23.3723) -> (94.25, -46.6277) projected
  arc A29 (94.25, -46.6277) -> (95.1071, -48.269) centre (96.25, -46.6277) ccw projected
  arc A30 (94.25, -51) -> (95.1071, -48.269) centre (94.25, -49.5) ccw projected
  line L90 (94.25, -51) -> (80.75, -51) projected
  arc A31 (79.8929, -48.269) -> (80.75, -51) centre (80.75, -49.5) ccw projected
  arc A32 (79.8929, -48.269) -> (80.75, -46.6277) centre (78.75, -46.6277) ccw projected
  line L91 (80.75, -46.6277) -> (80.75, -23.3723) projected
  arc A33 (-75.75, -11.6277) -> (-74.8929, -13.269) centre (-73.75, -11.6277) ccw projected
  arc A34 (-75.75, -16) -> (-74.8929, -13.269) centre (-75.75, -14.5) ccw projected
  line L92 (-75.75, -16) -> (-89.25, -16) projected
  arc A35 (-90.1071, -13.269) -> (-89.25, -16) centre (-89.25, -14.5) ccw projected
  arc A36 (-90.1071, -13.269) -> (-89.25, -11.6277) centre (-91.25, -11.6277) ccw projected
  line L93 (-89.25, -11.6277) -> (-89.25, 11.6277) projected
  arc A37 (-89.25, 11.6277) -> (-90.1071, 13.269) centre (-91.25, 11.6277) ccw projected
  arc A38 (-89.25, 16) -> (-90.1071, 13.269) centre (-89.25, 14.5) ccw projected
  line L94 (-89.25, 16) -> (-75.75, 16) projected
  arc A39 (-74.8929, 13.269) -> (-75.75, 16) centre (-75.75, 14.5) ccw projected
  arc A40 (-74.8929, 13.269) -> (-75.75, 11.6277) centre (-73.75, 11.6277) ccw projected
  line L95 (-75.75, 11.6277) -> (-75.75, -11.6277) projected
hole "Hole4" at (-105, 6.35, 105) at (-105, 6.35, 0) at (-105, 6.35, -105) at (0, 6.35, -105) at (110, 6.35, -105) at (110, 6.35, 0) at (110, 6.35, 105) at (0, 6.35, 105) at (0, 6.35, 0) direction (0, -1, 0) diameter 3.2 end through all clearance for "Socket Head Cap Screw" size "M3" standard "Ansi Metric M Profile"
sketch "Sketch24" plane through (0, 6.35, 0) normal (0, 1, 0) x (1, 0, 0)
  circle A0 centre (-1.5, 19.5) radius 1.5 projected
  circle A1 centre (-1.5, -19.5) radius 1.5 projected
  circle A2 centre (-1.5, -19.5) radius 1.2
  circle A3 centre (-1.5, 19.5) radius 1.2
  point P0 (0, 0)
  dimension "d108" = 2.4
  dimension "d109" = 2.4
  constraints: 2 centre point, 2 coincident
  measures "d108" diameter of A2
  measures "d109" diameter of A3
extrude "Extrusion13" add sketch "Sketch24" against normal up to surface (6.35 mm away)
body "Solid1"
